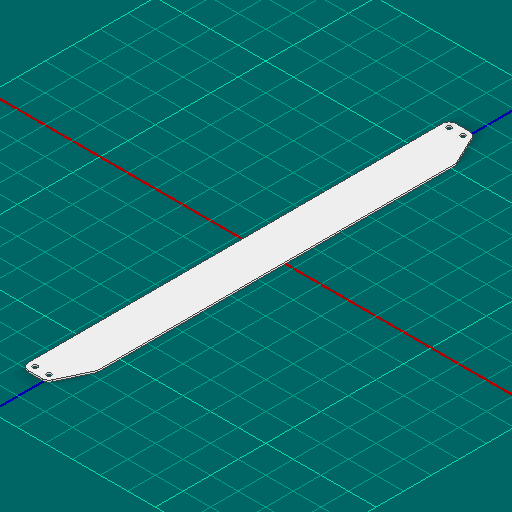
# Autodesk Inventor part: skirt
Saved by Autodesk Inventor 2025 (Build 290162000, 162)
## iProperties
Created: 2024-08-21
Part Number: skirt
Material: Acetal Resin, White
Document SubType Name: Modeling
Designer: averey
Density: 1.425 g/cm^3
Appearance: Smooth - White
Author: averey
Autodesk Inventor part; units mm, degrees
ref_plane "YZ Plane" through (0, 0, 0) normal (1, 0, 0) x (0, 1, 0)
ref_plane "XZ Plane" through (0, 0, 0) normal (0, 1, 0) x (-1, 0, 0)
ref_plane "XY Plane" through (0, 0, 0) normal (0, 0, 1) x (1, 0, 0)
sketch "Sketch1" plane through (0, 0, 0) normal (0, 1, 0) x (-1, 0, 0)
  circle A0 centre (0.6852, 198.77) radius 2.1844
  circle A1 centre (13.3852, 198.77) radius 2.1844
  circle A2 centre (13.3833, -182.23) radius 2.1844
  circle A3 centre (0.6833, -182.2338) radius 2.1844
  arc A4 (19.7352, 198.77) -> (13.3852, 205.12) centre (13.3852, 198.77) ccw
  arc A5 (0.6852, 205.12) -> (-5.0541, 201.487) centre (0.6852, 198.77) ccw
  arc A6 (13.3795, -188.5838) -> (19.7372, -182.23) centre (13.3833, -182.23) ccw
  arc A7 (-5.0525, -184.9492) -> (0.6814, -188.5799) centre (0.6833, -182.2338) ccw
  line L0 (13.3852, 205.12) -> (0.6852, 205.12)
  line L1 (13.3833, -188.5838) -> (0.6814, -188.5799)
  line L2 (19.7352, 198.77) -> (19.7372, -182.23)
  line L3 (-18.3648, 173.37) -> (-18.3648, -156.83)
  line L4 (-18.3648, -156.83) -> (-5.0525, -184.9492)
  line L5 (-18.3648, 173.37) -> (-5.0541, 201.487)
  point P0 (0, 0)
  dimension "d0" = 330.2
  constraints: 12 end point, 11 point on circle, 8 centre point, 7 tangent, 4 coincident, 3 point on line, 1 vertical, 1 other
  measures "d0" distance of L3.start L3.end
extrude "Extrusion1" add sketch "Sketch1" along normal blind 1.5875
body "Solid1"
